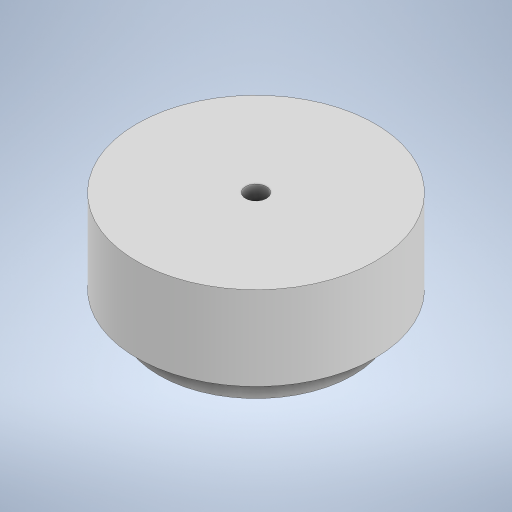
# Autodesk Inventor part: bottle
Saved by Autodesk Inventor 2023.1 (Build 271208000, 208)
## iProperties
Created: 2023-05-02
Part Number: bottle
Material: Generic
Document SubType Name: Modeling
Designer: dinesh
Density: 1 g/cm^3
Appearance: Default
Author: dinesh
Autodesk Inventor part; units mm, degrees
ref_plane "YZ Plane" through (0, 0, 0) normal (1, 0, 0) x (0, 1, 0)
ref_plane "XZ Plane" through (0, 0, 0) normal (0, 1, 0) x (-1, 0, 0)
ref_plane "XY Plane" through (0, 0, 0) normal (0, 0, 1) x (1, 0, 0)
sketch "Sketch1" plane through (0, 0, 0) normal (0, 0, 1) x (1, 0, 0)
  line L0 (2, 10) -> (22.75, 10)
  line L1 (22.75, 10) -> (22.75, 0)
  line L2 (2, 2) -> (2, 10)
  line L3 (0, 19.5472) -> (0, -22.4151)
  line L4 (22.75, 0) -> (21.75, 0) construction
  line L5 (21.75, 0) -> (21.75, -6)
  line L6 (21.75, -6) -> (22.75, -6)
  line L7 (22.75, -6) -> (22.75, 0)
  line L8 (20.25, 0) -> (17.5, 0) construction
  line L9 (17.5, -5) -> (17.5, -5)
  line L10 (17.5, -5) -> (20.25, -5) construction
  line L11 (20.25, -5) -> (20.25, 0)
  arc A0 (2, 2) -> (4, 0) centre (4, 2) ccw
  line L12 (21.75, 0) -> (20.25, 0)
  line L13 (12.5, 0) -> (4, 0)
  line L14 (-20.0393, 0) -> (21.75, 0) construction
  line L15 (22.75, 0) -> (24.5476, 0) construction
  arc A1 (17.5, -5) -> (12.5, 0) centre (12.5, -5) ccw
  line L16 (18.5, 0) -> (18.5, -5) construction
  line L17 (20.25, -5) -> (18.5, -5)
  line L18 (18.5, -5) -> (18.5, -11)
  line L19 (18.5, -11) -> (18.4, -11)
  line L20 (18.4, -11) -> (17.5, -5)
  point P0 (0, 0)
  dimension "d0" = 4
  dimension "d2" = 1
  dimension "d5" = 5
  dimension "d6" = 1.5
  dimension "d7" = 43.5
  dimension "d11" = 2
  dimension "d12" = 10
  dimension "d13" = 5
  dimension "d14" = 6
  dimension "d23" = 37
  dimension "d24" = 1
  dimension "d25" = 0.1
  dimension "d26" = 6
  constraints: 42 end point, 7 parallel, 7 point on line, 5 collinear, 5 horizontal, 5 perpendicular, 5 tangent, 4 point on circle, 2 centre point, 2 vertical
  measures "d0" diameter of L2 L3
  measures "d2" distance between parallel lines of L5 L7
  measures "d5" distance between parallel lines of L10 L8
  measures "d6" distance between parallel lines of L5 L11
  measures "d7" diameter of L5 L3
  measures "d11" radius of A0
  measures "d12" distance between parallel lines of L13 L0
  measures "d13" radius of A1
  measures "d14" distance between parallel lines of L6 L4
  measures "d23" diameter of L16 L3
  measures "d24" distance edge to line of A1 L16
  measures "d25" distance of L18.end L19.end
  measures "d26" distance between parallel lines of L19 L10
revolve "Revolution1" add sketch "Sketch1" angle 360 about axis through (0, 19.5472, 0) along (0, -1, 0)
sketch "Sketch2" plane through (0, 0, 0) normal (0, 0, 1) x (1, 0, 0)
  line L0 (-4, 0) -> (4, 0) projected
  line L1 (-2, 10) -> (2, 10) projected
  line L2 (0, 10) -> (0, 0) construction
  line L3 (-2, 2) -> (2, 2) construction
  circle A0 centre (0, 2.5) radius 2
  point P0 (1.9365, 2)
  point P1 (-1.9365, 2)
  dimension "d16" = 4
  dimension "d17" = 2.5
  constraints: 2 end point, 1 centre point, 1 midpoint, 1 perpendicular, 1 point on line
  measures "d16" diameter of A0
  measures "d17" distance from line of L0 A0.centre
extrude "Extrusion1" cut sketch "Sketch2" along normal blind 2 and the other way blind 32.625
equation "\"d0\" = t_D"
equation "\"d2\" = w_th"
equation "\"d5\" = b_rim_h"
equation "\"d6\" = lv_th"
equation "\"d7\" = b_OD"
equation "\"d11\" = fillet_D"
equation "\"d12\" = top_th_f"
equation "\"d13\" = 2.5 * fillet_D"
equation "\"d14\" = w_l"
equation "\"d23\" = b_ID"
equation "\"d24\" = w_th"
equation "\"d25\" = tol"
equation "\"d26\" = w_l"
equation "\"d16\" = t_D"
equation "\"d17\" = 0.5 * w_th + 0.5 * t_D"
equation "\"d18\" = 0.5 * t_D"
equation "\"d19\" = 0.75 * b_OD"
equation "\"tol\" = 0.1"
equation "\"fillet_D\" = 2"
equation "\"w_th\" = 1"
equation "\"w_l\" = 6"
equation "\"t_D\" = 4"
equation "\"t_D_f\" = t_D + w_th"
equation "\"top_th_f\" = t_D_f + cn_h"
equation "\"cn_h\" = 5"
equation "\"lv_th\" = 1.5"
equation "\"d3\" = w_l"
equation "\"b_ID\" = 37"
equation "\"b_OD\" = 43.5"
equation "\"b_rim_h\" = 5"
equation "\"top_th\" = t_D + w_th"
equation "\"lv_OD\" = 26"
equation "\"sv_OD\" = 13"
equation "\"sv_th\" = 1.5"
equation "\"b_th\" = 1.5"
body "Solid1"
